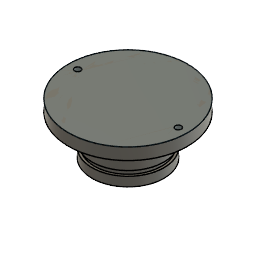
Robust_Cap_ScrewHoles (Autodesk Fusion 360 design; units mm, degrees)
part number: 2026-04-06-11-19-12-230
Autodesk Fusion 360 part; units mm, degrees
sketch "Sketch1" plane through (0, 0, 0) normal (0, 0, 1) x (1, 0, 0)
  line L0 (0, 0) -> (38.8, 0)
  line L1 (38.8, 0) -> (38.8, 10)
  line L2 (38.8, 10) -> (36.15, 10)
  line L3 (36.15, 10) -> (36.15, 15.3)
  line L4 (36.15, 15.3) -> (38.8, 15.3)
  line L5 (38.8, 15.3) -> (38.8, 27.3)
  line L6 (38.8, 27.3) -> (36.15, 27.3)
  line L7 (36.15, 27.3) -> (36.15, 32.6)
  line L8 (36.15, 32.6) -> (38.8, 32.6)
  line L9 (38.8, 32.6) -> (38.8, 42.6)
  line L10 (38.8, 42.6) -> (64.2, 42.6)
  line L11 (64.2, 42.6) -> (64.2, 55.3)
  line L12 (64.2, 55.3) -> (0, 55.3)
  line L13 (0, 55.3) -> (0, 0)
  dimension "d1" = 38.8
  dimension "d2" = 10
  dimension "d3" = 2.65
  dimension "d4" = 5.3
  dimension "d5" = 2.65
  dimension "d7" = 12
  dimension "d8" = 2.65
  dimension "d9" = 5.3
  dimension "d10" = 2.65
  dimension "d11" = 10
  dimension "d12" = 25.4
  dimension "d13" = 12.7
  constraint coincident L0.start L13.end
  constraint horizontal L0
  constraint perpendicular L0 L1
  constraint perpendicular L1 L2
  constraint perpendicular L2 L3
  constraint perpendicular L3 L4
  constraint perpendicular L4 L5
  constraint perpendicular L5 L6
  constraint perpendicular L6 L7
  constraint perpendicular L7 L8
  constraint perpendicular L8 L9
  constraint perpendicular L9 L10
  constraint perpendicular L10 L11
  constraint perpendicular L11 L12
  constraint perpendicular L0 L13
  measures "d1" distance of L0.start L0.end
  measures "d2" distance of L0.end L1.end
  measures "d3" distance of L1.end L2.end
  measures "d4" distance of L2.end L3.end
  measures "d5" distance of L3.end L4.end
  measures "d7" distance of L4.end L5.end
  measures "d8" distance of L5.end L6.end
  measures "d9" distance of L6.end L7.end
  measures "d10" distance of L7.end L8.end
  measures "d11" distance of L8.end L9.end
  measures "d12" distance of L9.end L10.end
  measures "d13" distance of L10.end L11.end
revolve "Revolve1" add sketch "Sketch1" angle 360 about axis through (0, 55.3, 0) along (0, -1, 0)
sketch "Sketch2" plane through (0, 55.3, 0) normal (0, 1, 0) x (-1, 0, 0)
  circle A0 centre (0, 0) radius 64.2
sketch "Sketch3" plane through (0, 55.3, 0) normal (0, 1, 0) x (-1, 0, 0)
  line L0 (-51.05, 0) -> (-54.25, 0)
  circle A0 centre (-54.25, 0) radius 3.2
  line L1 (51.05, 0) -> (54.25, 0)
  circle A1 centre (54.25, 0) radius 3.2
  dimension "d15" = 54.25
  dimension "d16" = 6.4
  dimension "d17" = 54.25
  dimension "d18" = 6.4
  constraint horizontal L0
  constraint coincident L0.end A0.centre
  constraint parallel L0 L1
  constraint coincident L1.end A1.centre
  constraint coincident A0 L0.start
  constraint coincident A1 L1.start
  measures "d15" distance of origin L0.end
  measures "d16" diameter of A0
  measures "d17" distance of origin L1.end
  measures "d18" diameter of A1
hole "Hole1" at (54.25, 55.3, 0) direction (0, -1, 0) diameter 6.4 depth 100 tip angle 118
sketch "Sketch4" plane through (0, 55.3, 0) normal (0, 1, 0) x (-1, 0, 0)
  line L0 (51.05, 0) -> (54.25, 0)
  circle A0 centre (54.25, 0) radius 3.2
  dimension "d22" = 54.25
  dimension "d23" = 6.4
  constraint horizontal L0
  constraint coincident L0.end A0.centre
  constraint coincident A0 L0.start
  measures "d22" distance of origin L0.end
  measures "d23" diameter of A0
hole "Hole2" at (-54.25, 55.3, 0) direction (0, -1, 0) diameter 6.4 depth 100 tip angle 118
